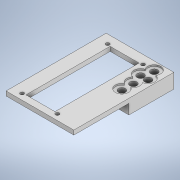
# Autodesk Inventor part: Button_Plate
Saved by Autodesk Inventor 2021 (Build 250183000, 183)
## iProperties
Created: 2021-07-06
Part Number: Button_Plate
Material: Generic
Document SubType Name: Modeling
Designer: rquic
Density: 1 g/cm^3
Appearance: Default
Author: rquic
Autodesk Inventor part; units mm, degrees
ref_plane "YZ Plane" through (0, 0, 0) normal (1, 0, 0) x (0, 1, 0)
ref_plane "XZ Plane" through (0, 0, 0) normal (0, 1, 0) x (-1, 0, 0)
ref_plane "XY Plane" through (0, 0, 0) normal (0, 0, 1) x (1, 0, 0)
sketch "Sketch1" plane through (0, 0, 0) normal (0, 1, 0) x (-1, 0, 0)
  line L0 (-24.384, 42.545) -> (24.384, 42.545)
  line L1 (24.384, 42.545) -> (24.384, -42.545)
  line L2 (24.384, -42.545) -> (-24.384, -42.545)
  line L3 (-24.384, -42.545) -> (-24.384, 42.545)
  line L4 (-24.384, 42.545) -> (24.384, -42.545) construction
  line L5 (24.384, 42.545) -> (-24.384, -42.545) construction
  line L6 (-12.7, 36.83) -> (12.7, 36.83)
  line L7 (12.7, 36.83) -> (12.7, -36.83)
  line L8 (12.7, -36.83) -> (-12.7, -36.83)
  line L9 (-12.7, -36.83) -> (-12.7, 36.83)
  line L10 (-12.7, 36.83) -> (12.7, -36.83) construction
  line L11 (12.7, 36.83) -> (-12.7, -36.83) construction
  line L12 (-24.384, 42.545) -> (-34.925, 42.545)
  line L13 (-34.925, 42.545) -> (-34.925, -42.545)
  line L14 (-34.925, -42.545) -> (-24.384, -42.545)
  line L15 (-24.384, -42.545) -> (-24.384, 42.545)
  circle A0 centre (15.494, 37.465) radius 1.5875
  circle A1 centre (-15.494, 37.465) radius 1.5875
  circle A2 centre (-15.494, -37.465) radius 1.5875
  circle A3 centre (15.494, -37.465) radius 1.5875
  point P0 (0, 0)
  dimension "d37" = 11.43
  dimension "d0" = 73.66
  dimension "d1" = 25.4
  dimension "d4" = 85.09
  dimension "d5" = 34.925
  dimension "d6" = 59.309
  dimension "d7" = 3.175
  dimension "d8" = 3.175
  dimension "d9" = 3.175
  dimension "d10" = 3.175
  dimension "d11" = 5.08
  dimension "d12" = 8.89
  dimension "d13" = 5.08
  dimension "d14" = 19.431
  constraints: 32 end point, 6 parallel, 4 centre point, 4 midpoint, 3 horizontal, 3 perpendicular, 2 horizontal alignment, 2 vertical alignment, 1 collinear
  measures "d0" distance of L6.end L7.end
  measures "d1" distance of L7.end L8.end
  measures "d4" distance between parallel lines of L2 L0
  measures "d5" distance from line of L13 point (0, 0)
  measures "d6" distance between parallel lines of L1 L13
  measures "d7" diameter of A3
  measures "d8" diameter of A2
  measures "d9" diameter of A1
  measures "d10" diameter of A0
  measures "d11" distance from line of L0 A0.centre
  measures "d12" distance from line of L1 A0.centre
  measures "d13" distance from line of L2 A2.centre
  measures "d14" distance from line of L13 A2.centre
extrude "Extrusion1" add sketch "Sketch1" along normal blind 3.81
sketch "Sketch3" plane through (0, 0, 0) normal (0, -1, 0) x (1, 0, 0)
  line L0 (34.925, 42.545) -> (34.925, -42.545) projected
  line L1 (34.925, -42.545) -> (17.78, -42.545)
  line L2 (17.78, -42.545) -> (17.78, -5.715)
  line L3 (17.78, -5.715) -> (34.925, -5.715)
  line L4 (34.925, -5.715) -> (34.925, -42.545)
  point P0 (0, 0)
  point P1 (34.925, -5.715)
  dimension "d31" = 36.83
  dimension "d32" = 17.145
  constraints: 8 end point, 2 parallel, 1 horizontal, 1 perpendicular
  measures "d31" distance of L1.end L2.end
  measures "d32" distance of L0.end L1.end
extrude "Extrusion3" add sketch "Sketch3" along normal blind 8.89
sketch "Sketch2" plane through (0, 3.81, 0) normal (0, 1, 0) x (1, 0, 0)
  circle A0 centre (21.59, 29.21) radius 3.0162
  circle A1 centre (28.194, 29.21) radius 3.0162
  circle A2 centre (24.638, 38.1) radius 3.0162
  circle A3 centre (24.638, 19.812) radius 3.0162
  line L0 (34.925, -42.545) -> (34.925, 42.545) projected
  circle A4 centre (24.638, 9.8298) radius 3.0162
  line L1 (34.925, 42.545) -> (-24.384, 42.545) projected
  point P0 (0, 0)
  dimension "d17" = 6.0325
  dimension "d18" = 6.0325
  dimension "d19" = 6.0325
  dimension "d20" = 6.0325
  dimension "d21" = 6.731
  dimension "d22" = 10.287
  dimension "d23" = 13.335
  dimension "d24" = 6.0325
  dimension "d25" = 4.445
  dimension "d26" = 18.288
  dimension "d27" = 8.89
  dimension "d28" = 28.2702
  constraints: 5 centre point, 2 vertical alignment, 1 horizontal alignment
  measures "d17" diameter of A2
  measures "d18" diameter of A0
  measures "d19" diameter of A3
  measures "d20" diameter of A1
  measures "d21" distance from line of L0 A1.centre
  measures "d22" distance from line of L0 A3.centre
  measures "d23" distance from line of L0 A0.centre
  measures "d24" diameter of A4
  measures "d25" distance from line of L1 A2.centre
  measures "d26" distance of A3.centre A2.centre
  measures "d27" vertical distance of A2.centre A0.centre
  measures "d28" distance of A4.centre A2.centre
extrude "Extrusion2" cut sketch "Sketch2" against normal through all
sketch "Sketch7" plane through (-24.384, 0, -42.545) normal (0, 0, -1) x (-1, 0, 0)
  line L0 (-59.309, 3.81) -> (0, 3.81) projected
  line L1 (0, 0) -> (-59.309, 0) projected
  line L2 (0, 3.81) -> (-59.309, 3.81)
  line L3 (-59.309, 3.81) -> (-59.309, 0)
  line L4 (-59.309, 0) -> (0, 0)
  line L5 (0, 0) -> (0, 3.81)
  line L6 (-42.164, -8.89) -> (-59.309, -8.89) projected
  line L7 (-59.309, -8.89) -> (-42.164, -8.89)
  line L8 (-42.164, -8.89) -> (-42.164, 0)
  line L9 (-42.164, 0) -> (-59.309, 0)
  line L10 (-59.309, 0) -> (-59.309, -8.89)
  point P0 (-24.384, 0)
  point P1 (-45.4299, 3.81)
  point P2 (-45.4299, 3.81)
  constraints: 16 end point, 4 parallel, 2 horizontal, 2 perpendicular, 1 point on line
extrude "Extrusion5" add sketch "Sketch7" along normal blind 2.54
sketch "Sketch4" plane through (0, 3.81, 0) normal (0, 1, 0) x (1, 0, 0)
  circle A0 centre (21.59, 29.21) radius 3.0162 projected
  circle A1 centre (21.59, 29.21) radius 5.715
  circle A2 centre (24.638, 38.1) radius 3.0162 projected
  circle A3 centre (24.638, 38.1) radius 5.715
  circle A4 centre (28.194, 29.21) radius 3.0162 projected
  circle A5 centre (24.638, 19.812) radius 3.0162 projected
  circle A6 centre (24.638, 19.812) radius 5.715
  circle A7 centre (24.638, 9.8298) radius 3.0162 projected
  circle A8 centre (24.638, 9.8298) radius 5.715
  circle A9 centre (28.194, 29.21) radius 5.715
  point P0 (0, 0)
  point P1 (24.892, 24.5455)
  point P2 (24.892, 33.8745)
  point P3 (23.8684, 25.4749)
  point P4 (23.108, 26.6036)
  point P5 (23.108, 31.8164)
  point P6 (23.518, 32.4958)
  point P7 (20.037, 34.71)
  point P8 (20.3805, 23.6245)
  point P9 (28.9636, 23.5471)
  point P10 (29.314, 34.8142)
  point P11 (26.191, 32.6)
  point P12 (26.676, 31.8164)
  point P13 (26.676, 26.6036)
  point P14 (25.8475, 25.3975)
  point P15 (21.8541, 14.8209)
  point P16 (27.4219, 14.8209)
  dimension "d35" = 11.43
  dimension "d36" = 11.43
  dimension "d37" = 11.43
  dimension "d38" = 11.43
  dimension "d39" = 11.43
  constraints: 5 centre point, 5 coincident
  measures "d35" diameter of A3
  measures "d36" diameter of A9
  measures "d37" diameter of A1
  measures "d38" diameter of A6
  measures "d39" diameter of A8
extrude "Extrusion6" cut sketch "Sketch4" against normal blind 1.27 contours A0 A9 A3 A1 A4 A6 | A0 A9 A6 A1 A3 | A9 A1 A3 | A3 A1 A9 | A9 A1 A6 | A6 A1 A9 | A3 A9 A1 | A3 A9 A6 A1 A4 | A1 A9 A3 | A6 A9 A1 | A1 A9 A6 A8 | A8 A6 | A6 A8
equation "\"d37\" = d35"
equation "\"d8\" = d7"
equation "\"d9\" = d7"
equation "\"d10\" = d7"
equation "\"d18\" = d17"
equation "\"d19\" = d17"
equation "\"d20\" = d17"
equation "\"d24\" = d17"
equation "\"d36\" = d35"
equation "\"d38\" = d35"
equation "\"d39\" = d35"
body "Solid1"
